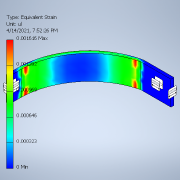
# Autodesk Inventor part: UHMWBMockup
Saved by Autodesk Inventor 2021 (Build 250183000, 183)
## iProperties
Created: 2021-04-14
Part Number: UHMWBMockup
Material: UHMW, White
Document SubType Name: Modeling
Designer: Esketitttttt
Density: 0.94 g/cm^3
Appearance: Smooth - White
Author: Esketitttttt
Autodesk Inventor part; units mm, degrees
ref_plane "YZ Plane" through (0, 0, 0) normal (1, 0, 0) x (0, 1, 0)
ref_plane "XZ Plane" through (0, 0, 0) normal (0, 1, 0) x (-1, 0, 0)
ref_plane "XY Plane" through (0, 0, 0) normal (0, 0, 1) x (1, 0, 0)
sketch "Sketch1" plane through (0, 0, 0) normal (0, 1, 0) x (-1, 0, 0)
  line L0 (0, 0) -> (235.3817, 0) construction
  line L1 (235.3817, 0) -> (235.3817, -328.93) construction
  line L2 (235.3817, -328.93) -> (0, -328.93) construction
  line L3 (0, -328.93) -> (0, 0) construction
  line L4 (235.3817, 0) -> (222.6817, 0)
  line L5 (0, -328.93) -> (0, -341.63) construction
  line L6 (222.6817, 0) -> (222.6817, -50.8)
  line L7 (235.3817, 0) -> (235.3817, -50.8)
  arc A0 (0, -328.93) -> (222.6817, -50.8) centre (-67.6135, -46.5872) ccw
  arc A1 (0, -341.63) -> (235.3817, -50.8) centre (-61.9792, -50.8) ccw
  line L8 (222.6817, -50.8) -> (235.3817, -50.8) construction
  line L9 (0, -328.93) -> (-127, -328.93)
  line L10 (-127, -328.93) -> (-127, -341.63)
  line L11 (-127, -341.63) -> (0, -341.63)
  line L12 (0, -341.63) -> (0, -328.93) construction
  point P0 (0, -341.63)
  dimension "d0" = 235.3817
  dimension "d1" = 328.93
  dimension "t" = 12.7
  dimension "d3" = 12.7
  dimension "d4" = 50.8
  dimension "d5" = 127
  dimension "d6" = 12.7
  constraints: 26 end point, 4 parallel, 4 point on circle, 3 horizontal, 2 centre point, 2 perpendicular, 2 point on line, 2 tangent, 2 vertical
  measures "d0" distance of L1.end L2.end
  measures "d1" distance of L0.end L1.end
  measures "t" distance of L0.end L4.end
  measures "d3" distance of L2.end L5.end
  measures "d4" distance of L4.end L6.end
  measures "d5" distance of L11.end L10.end
  measures "d6" distance of L9.end L10.end
extrude "Extrusion1" add sketch "Sketch1" along normal blind 101.6
equation "\"d3\" = t"
equation "\"d6\" = t"
body "Solid1"
